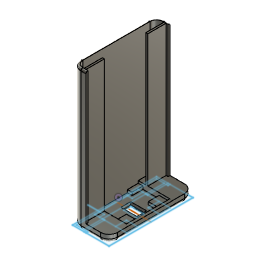
People Counter Pololu (Autodesk Fusion 360 design; units mm, degrees)
Autodesk Fusion 360 part; units mm, degrees
sketch "Skizze1" plane through (0, 0, 0) normal (0, 0, 1) x (1, 0, 0)
  line L0 (5.7561, -0.6264) -> (11.1561, -0.6264)
  line L1 (11.1561, -0.6264) -> (11.1561, -3.5264)
  line L2 (11.1561, -3.5264) -> (5.7561, -3.5264)
  line L3 (5.7561, -3.5264) -> (5.7561, -0.6264)
  line L4 (0.4561, 15.4236) -> (15.6561, 15.4236)
  line L5 (15.6561, 15.4236) -> (15.6561, -19.5764)
  line L6 (15.6561, -19.5764) -> (0.4561, -19.5764)
  line L7 (0.4561, -19.5764) -> (0.4561, 15.4236)
  line L8 (11.1561, -2.0764) -> (5.7561, -2.0764) construction
  line L9 (1.2561, 14.6236) -> (4.4561, 14.6236)
  line L10 (4.4561, 14.6236) -> (4.4561, -18.7764)
  line L11 (4.4561, -18.7764) -> (1.2561, -18.7764)
  line L12 (1.2561, -18.7764) -> (1.2561, 14.6236)
  line L13 (4.4561, 6.9236) -> (5.2561, 6.9236)
  line L14 (5.2561, 6.9236) -> (5.2561, 15.4236)
  line L15 (4.4561, -11.0764) -> (5.2561, -11.0764)
  line L16 (5.2561, -11.0764) -> (5.2561, -19.5764)
  line L17 (5.2561, 14.6236) -> (6.0561, 14.6236)
  line L18 (6.0561, 14.6236) -> (6.0561, 15.4236)
  line L19 (5.2561, -18.7764) -> (6.0561, -18.7764)
  line L20 (6.0561, -18.7764) -> (6.0561, -19.5764)
  line L21 (1.2561, -11.1264) -> (14.4561, -11.1264)
  line L22 (14.4561, -11.1264) -> (14.4561, 6.9736)
  line L23 (14.4561, 6.9736) -> (1.2561, 6.9736)
  line L24 (1.2561, 6.9736) -> (1.2561, -11.1264)
  line L25 (14.4561, -2.0764) -> (1.2561, -2.0764) construction
  line L26 (15.6561, -2.0764) -> (0.4561, -2.0764) construction
  line L27 (3.2561, 6.9736) -> (3.2561, 2.4736)
  line L28 (3.2561, 2.4736) -> (1.2561, 2.4736)
  line L29 (1.2561, -9.1264) -> (-3.5583, -9.1264)
  line L30 (-3.5583, -9.1264) -> (3.2561, -9.1264)
  line L31 (3.2561, -9.1264) -> (3.2561, -11.1264)
  line L32 (9.9561, -11.1264) -> (9.9561, -6.6264)
  line L33 (9.9561, -6.6264) -> (14.4561, -6.6264)
  line L34 (9.9561, 6.9736) -> (9.9561, 2.4736)
  line L35 (9.9561, 2.4736) -> (14.4561, 2.4736)
  dimension "d7" = 5.4
  dimension "d8" = 2.9
  dimension "d42" = 35
  dimension "d45" = 0.8
  dimension "d46" = 0.8
  dimension "d47" = 0.8
  dimension "d48" = 3.2
  dimension "d51" = 8.5
  dimension "d52" = 8.5
  dimension "d53" = 0.8
  dimension "d55" = 0.8
  dimension "d56" = 0.8
  dimension "d57" = 0.8
  dimension "d58" = 0.8
  dimension "d70" = 18.1
  dimension "d71" = 13.2
  dimension "d72" = 3.3
  dimension "d73" = 1.2
  dimension "d75" = 2
  dimension "d76" = 4.5
  dimension "d77" = 2
  dimension "d79" = 4.5
  dimension "d80" = 4.5
  dimension "d81" = 4.5
  constraint horizontal L0
  constraint vertical L1
  constraint horizontal L2
  constraint vertical L3
  constraint horizontal L4
  constraint vertical L5
  constraint horizontal L6
  constraint vertical L7
  constraint midpoint L1 L8.start
  constraint midpoint L3 L8.end
  constraint horizontal L9
  constraint vertical L10
  constraint horizontal L11
  constraint vertical L12
  constraint coincident L10 L13.start
  constraint perpendicular L10 L13
  constraint coincident L4 L14.end
  constraint perpendicular L4 L14
  constraint coincident L10 L15.start
  constraint perpendicular L10 L15
  constraint coincident L6 L16.end
  constraint perpendicular L6 L16
  constraint collinear L14 L16
  constraint coincident L14 L17.start
  constraint perpendicular L14 L17
  constraint coincident L4 L18.end
  constraint perpendicular L4 L18
  constraint coincident L16 L19.start
  constraint perpendicular L16 L19
  constraint coincident L6 L20.end
  constraint perpendicular L6 L20
  constraint horizontal L21
  constraint vertical L22
  constraint horizontal L23
  constraint vertical L24
  constraint midpoint L22 L25.start
  constraint midpoint L24 L25.end
  constraint collinear L8 L25
  constraint midpoint L5 L26.start
  constraint midpoint L7 L26.end
  constraint collinear L25 L26
  constraint collinear L12 L24
  constraint coincident L23 L27.start
  constraint perpendicular L23 L27
  constraint coincident L24 L28.end
  constraint coincident L12 L29.start
  constraint perpendicular L12 L29
  constraint perpendicular L12 L30
  constraint coincident L21 L31.end
  constraint perpendicular L21 L31
  constraint perpendicular L24 L28
  constraint coincident L21 L32.start
  constraint perpendicular L21 L32
  constraint coincident L22 L33.end
  constraint perpendicular L22 L33
  constraint coincident L23 L34.start
  constraint perpendicular L23 L34
  constraint coincident L22 L35.end
  constraint perpendicular L22 L35
  constraint collinear L32 L34
  constraint collinear L27 L31
  measures "d7" distance of L0.start L0.end
  measures "d8" distance of L0.start L2.end
  measures "d42" distance of L4.start L6.end
  measures "d45" distance of L6 L11
  measures "d46" distance of L4 L9
  measures "d47" distance of L7 L12
  measures "d48" distance of L10 L12
  measures "d51" distance of L13.end L14.end
  measures "d52" distance of L15.end L16.end
  measures "d53" distance of L10 L16
  measures "d55" distance of L19.start L19.end
  measures "d56" distance of L19.end L20.end
  measures "d57" distance of L17.end L18.end
  measures "d58" distance of L14 L18
  measures "d70" distance of L21.end L22.end
  measures "d71" distance of L22.end L23.end
  measures "d72" distance of L1 L22
  measures "d73" distance of L5 L22
  measures "d75" distance of L30.end L31.end
  measures "d76" distance of L27.start L27.end
  measures "d77" distance of L27.end L28.end
  measures "d79" distance of L32.end L33.end
  measures "d80" distance of L34.start L34.end
  measures "d81" distance of L32.start L32.end
extrude "Extrusion1" add sketch "Skizze1" along normal blind 1 contours L12 L21 L24 L30 L31 | L10 L12 L21 L23 L24 L27 L28 L30 L31 | L10 L13 L14 L15 L16 L21 L22 L23 L32 L33 L34 L35 | L10 L13 L14 L23 | L12 L23 L24 L27 L28 | L22 L23 L34 L35 | L10 L15 L16 L21 | L21 L22 L32 L33
extrude "Extrusion5" add sketch "Skizze1" along normal blind 2.2 contours L12 L21 L24 L30 L31 | L12 L23 L24 L27 L28 | L22 L23 L34 L35 | L21 L22 L32 L33
extrude "Extrusion2" add sketch "Skizze1" along normal blind 3.2 contours L4 L7 L9 L10 L12 L14 L23 L24 L29 L30 | L4 L14 L17 L18 | L6 L7 L10 L11 L12 L16 L21 L24 L29 L30 | L4 L5 L6 L14 L16 L17 L18 L19 L20 L21 L22 L23 | L6 L16 L19 L20 | L10 L11 L12 L21 | L9 L10 L12 L23
extrude "Extrusion4" add sketch "Skizze1" along normal blind 55 from surface at 3.2 contours L4 L7 L9 L10 L12 L14 L23 L24 L29 L30 | L4 L14 L17 L18 | L6 L7 L10 L11 L12 L16 L21 L24 L29 L30 | L6 L16 L19 L20
fillet "Abrundung1" radius 2.7 2 edges at (1.2561, 14.6236, 30.7) (1.2561, -18.7764, 30.7)
fillet "Abrundung2" radius 1.5 4 edges at (0.4561, -2.0764, 0) (8.0561, 15.4236, 0) (8.0561, -19.5764, 0) (15.6561, -2.0764, 0)
fillet "Abrundung4" radius 3.5 8 edges at (0.8955, -19.1371, 0.4393) (0.4561, -19.5764, 29.85) (0.8955, 14.9843, 0.4393) (0.4561, 15.4236, 29.85) (15.2168, 14.9843, 0.4393) (15.6561, 15.4236, 2.35) (15.2168, -19.1371, 0.4393) (15.6561, -19.5764, 2.35)
fillet "Abrundung3" radius 0.8 5 edges at (5.0061, -19.5764, 58.2) (1.4812, -18.5513, 58.2) (0.4561, -2.0764, 58.2) (1.4812, 14.3985, 58.2) (5.0061, 15.4236, 58.2)
chamfer "Fase2" distance 0.6 angle 45 4 edges at (8.4561, -0.6264, 1) (5.7561, -2.0764, 1) (8.4561, -3.5264, 1) (11.1561, -2.0764, 1)
equation "d27 = 1 mm + 1.2 mm + 1 mm"
equation "d51 = ( ( 35 - 18 ) / 2 ) * 1 mm"
equation "d52 = ( ( 35 - 18 ) / 2 ) * 1 mm"
equation "d61 = 3.5 mm - 0.8 mm"
equation "d68 = 1 mm + 1.2 mm + 1 mm"
equation "d82 = 1 mm + 1.2 mm"
named bodies: "Person_Tracker"
